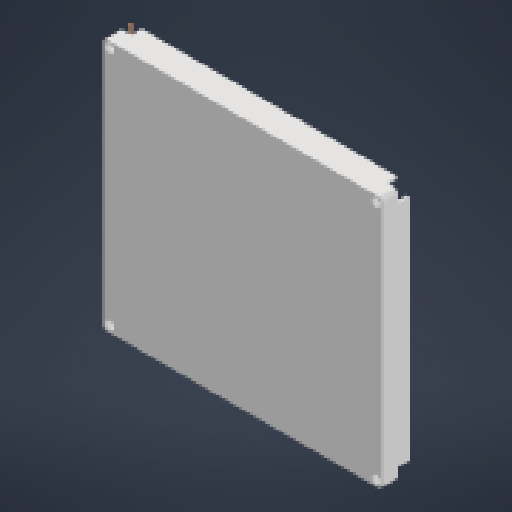
# Autodesk Inventor part: tutup_box_alert
Saved by Autodesk Inventor 2027.1 (Build 311270010, 270A)
## iProperties
Created: 2026-09-21
Part Number: tutup_box_alert
Material: Generic
Document SubType Name: Modeling
Designer: LENOVO
Density: 1 g/cm^3
Appearance: Default
Author: LENOVO
Autodesk Inventor part; units mm, degrees
ref_plane "YZ Plane" through (0, 0, 0) normal (1, 0, 0) x (0, 1, 0)
ref_plane "XZ Plane" through (0, 0, 0) normal (0, 1, 0) x (-1, 0, 0)
ref_plane "XY Plane" through (0, 0, 0) normal (0, 0, 1) x (1, 0, 0)
sketch "Sketch1" plane through (0, 0, 0) normal (0, 0, 1) x (1, 0, 0)
  arc A0 (47.5, 45) -> (50, 42.5) centre (49.4114, 44.4114) ccw projected
  line L0 (50, 42.5) -> (50, -42.5) projected
  arc A1 (50, -42.5) -> (47.5, -45) centre (49.4114, -44.4114) ccw projected
  line L1 (47.5, -45) -> (-47.5, -45) projected
  arc A2 (-47.5, -45) -> (-50, -42.5) centre (-49.4114, -44.4114) ccw projected
  line L2 (-50, -42.5) -> (-50, 42.5) projected
  arc A3 (-50, 42.5) -> (-47.5, 45) centre (-49.4114, 44.4114) ccw projected
  line L3 (-47.5, 45) -> (47.5, 45) projected
  circle A4 centre (-49.6464, 44.6464) radius 1.35 projected
  circle A5 centre (-49.6464, -44.6464) radius 1.35 projected
  circle A6 centre (49.6464, -44.6464) radius 1.35 projected
  circle A7 centre (49.6464, 44.6464) radius 1.35 projected
  arc A8 (-52, -45.5) -> (-50.5, -47) centre (-50.5, -45.5) ccw projected
  line L4 (-50.5, -47) -> (-47.5, -47) projected
  line L5 (-47.5, -47) -> (-47.5, -46) projected
  line L6 (-47.5, -46) -> (47.5, -46) projected
  line L7 (47.5, -46) -> (47.5, -47) projected
  line L8 (47.5, -47) -> (50.5, -47) projected
  arc A9 (50.5, -47) -> (52, -45.5) centre (50.5, -45.5) ccw projected
  line L9 (52, -45.5) -> (52, -42.5) projected
  line L10 (52, -42.5) -> (51, -42.5) projected
  line L11 (51, -42.5) -> (51, 42.5) projected
  line L12 (51, 42.5) -> (52, 42.5) projected
  line L13 (52, 42.5) -> (52, 45.5) projected
  arc A10 (52, 45.5) -> (50.5, 47) centre (50.5, 45.5) ccw projected
  line L14 (50.5, 47) -> (47.5, 47) projected
  line L15 (47.5, 47) -> (47.5, 46) projected
  line L16 (47.5, 46) -> (-47.5, 46) projected
  line L17 (-47.5, 46) -> (-47.5, 47) projected
  line L18 (-47.5, 47) -> (-50.5, 47) projected
  arc A11 (-50.5, 47) -> (-52, 45.5) centre (-50.5, 45.5) ccw projected
  line L19 (-52, 45.5) -> (-52, 42.5) projected
  line L20 (-52, 42.5) -> (-51, 42.5) projected
  line L21 (-51, 42.5) -> (-51, -42.5) projected
  line L22 (-51, -42.5) -> (-52, -42.5) projected
  line L23 (-52, -42.5) -> (-52, -45.5) projected
  point P0 (0, 0)
extrude "Extrusion1" add sketch "Sketch1" along normal blind 6
ref_plane "Work Plane1" through (-51.5, 0, -4) normal (0, 0, 1) x (1, 0, 0)
sketch "Sketch2" plane through (-51.5, 0, -4) normal (0, 0, 1) x (1, 0, 0)
  line L0 (99, 47) -> (99, 46) projected
  line L1 (4, 47) -> (99, 47) projected
  line L2 (4, 46) -> (4, 47) projected
  line L3 (99, 46) -> (4, 46) projected
  line L4 (-0.5, 42.5) -> (0.5, 42.5) projected
  line L5 (-0.5, -42.5) -> (-0.5, 42.5) projected
  line L6 (0.5, -42.5) -> (-0.5, -42.5) projected
  line L7 (0.5, 42.5) -> (0.5, -42.5) projected
  line L8 (103.5, -42.5) -> (102.5, -42.5) projected
  line L9 (103.5, 42.5) -> (103.5, -42.5) projected
  line L10 (102.5, 42.5) -> (103.5, 42.5) projected
  line L11 (102.5, -42.5) -> (102.5, 42.5) projected
  line L12 (4, -47) -> (4, -46) projected
  line L13 (99, -47) -> (4, -47) projected
  line L14 (99, -46) -> (99, -47) projected
  line L15 (4, -46) -> (99, -46) projected
  point P0 (51.5, 0)
extrude "Extrusion2" add sketch "Sketch2" along normal blind 10
sketch "Sketch3" plane through (-52, -45.5, 6) normal (-1, 0, 0) x (0, 0, 1)
  line L0 (-6, 91) -> (-6, 88) projected
  line L1 (-10, 88) -> (-6, 88) projected
  line L2 (-10, 88) -> (-10, 3) projected
  line L3 (-10, 3) -> (-6, 3) projected
  line L4 (-6, 3) -> (-6, 0) projected
  line L5 (-6, 0) -> (0, 0) projected
  line L6 (0, 91) -> (0, 0) projected
  line L7 (-6, 91) -> (0, 91) projected
  line L8 (-6, 92.5) -> (0, 92.5) projected
  line L9 (0, 91) -> (0, 92.5) projected
  line L10 (-6, 92.5) -> (-6, 91) projected
  line L11 (-6, 91) -> (0, 91) projected
  line L12 (0, 92.5) -> (0, 91) projected
  line L13 (-6, 92.5) -> (0, 92.5) projected
  line L14 (-6, -1.5) -> (0, -1.5) projected
  line L15 (0, -1.5) -> (0, 0) projected
  line L16 (0, 92.5) -> (-2, 92.5)
  line L17 (-2, 92.5) -> (-2, -1.5)
  line L18 (-2, -1.5) -> (0, -1.5)
  line L19 (0, -1.5) -> (0, 92.5)
  point P0 (-6, 45.5)
  dimension "d4" = 2
  constraints: 8 end point, 2 parallel, 1 horizontal, 1 perpendicular, 1 point on line
  measures "d4" distance of L18.end L17.end
extrude "Extrusion3" add sketch "Sketch3" against normal blind 104 contours L17 L8 L9 L7 | L7 L6 L5 L17 | L5 L15 L14 L17
fillet "Fillet1" radius 1.5 4 edges at (-52, -47, 5) (-52, 47, 5) (52, 47, 5) (52, -47, 5)
sketch "Sketch4" plane through (0, 0, 6) normal (0, 0, 1) x (1, 0, 0)
  circle A0 centre (49.6464, -44.6464) radius 1.35 projected
  circle A1 centre (-49.6464, -44.6464) radius 1.35 projected
  circle A2 centre (-49.6464, 44.6464) radius 1.35 projected
  circle A3 centre (49.6464, 44.6464) radius 1.35 projected
  point P0 (0, 0)
hole "Hole1" at (49.6464, 44.6464, 6) at (-49.6464, 44.6464, 6) at (-49.6464, -44.6464, 6) at (49.6464, -44.6464, 6) direction (0, 0, -1) diameter 2.7 depth 10 tip angle 118 countersink diameter 3.5 countersink angle 90
body "Solid1"
